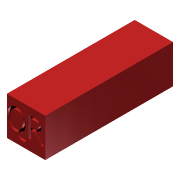
# Autodesk Inventor part: Container 2 2 5 QR color 5
Saved by Autodesk Inventor 2015 (Build 190159000, 159)
## iProperties
Created: 2015-03-07
Part Number: Container 2 2 5 QR color 5
Material: Generic
Document SubType Name: Modeling
Designer: Vukica
Density: 1 g/cm^3
Appearance: Light Red
Author: Vukica
Autodesk Inventor part; units mm, degrees
ref_plane "YZ Plane" through (0, 0, 0) normal (1, 0, 0) x (0, 1, 0)
ref_plane "XZ Plane" through (0, 0, 0) normal (0, 1, 0) x (-1, 0, 0)
ref_plane "XY Plane" through (0, 0, 0) normal (0, 0, 1) x (1, 0, 0)
sketch "Sketch1" plane through (0, 0, 0) normal (0, 0, 1) x (1, 0, 0)
  line L0 (0, 0) -> (38.1, 0)
  line L1 (38.1, 0) -> (38.1, 38.1)
  line L2 (38.1, 38.1) -> (0, 38.1)
  line L3 (0, 38.1) -> (0, 0)
  dimension "d0" = 38.1
  dimension "d1" = 38.1
  constraints: 8 end point, 2 parallel, 1 horizontal, 1 perpendicular
  measures "d0" distance of L1.end L2.end
  measures "d1" distance of L2.end L0.start
extrude "Extrusion1" add sketch "Sketch1" along normal blind 127
sketch "Sketch2" plane through (0, 0, 127) normal (0, 0, 1) x (1, 0, 0)
  line L0 (-0.4591, 31.2765) -> (45.936, 31.2765) construction
  line L1 (45.936, 31.2765) -> (45.936, -1.3483) construction
  line L2 (45.936, -1.3483) -> (-0.4591, -1.3483) construction
  line L3 (-0.4591, -1.3483) -> (-0.4591, 31.2765) construction
  spline S0 degree 2 poles (18.4777, 5.5554) (17.7367, 5.3742) (16.1229, 5.1766) (15.3161, 5.1766) knots 0 0 0 1 2 2 2
  spline S1 degree 2 poles (15.3161, 5.1766) (13.0272, 5.1766) (10.1784, 7.729) (10.0467, 10.1002) knots 0 0 0 1 2 2 2
  spline S2 degree 2 poles (10.0467, 10.1002) (9.8656, 10.1002) (9.5527, 10.1002) (9.421, 10.1002) knots 0 0 0 1 2 2 2
  spline S3 degree 2 poles (9.421, 10.1002) (7.3626, 10.1002) (4.0528, 11.4999) (2.8672, 12.8666) knots 0 0 0 1 2 2 2
  spline S4 degree 2 poles (2.8672, 12.8666) (1.698, 14.2169) (0.4466, 18.1689) (0.4466, 20.6719) knots 0 0 0 1 2 2 2
  spline S5 degree 2 poles (0.4466, 20.6719) (0.4466, 23.2407) (1.7145, 27.1269) (2.8837, 28.5101) knots 0 0 0 1 2 2 2
  spline S6 degree 2 poles (2.8837, 28.5101) (4.0693, 29.8768) (7.3791, 31.2765) (9.421, 31.2765) knots 0 0 0 1 2 2 2
  spline S7 degree 2 poles (9.421, 31.2765) (11.4958, 31.2765) (14.8221, 29.8274) (15.9747, 28.5101) knots 0 0 0 1 2 2 2
  spline S8 degree 2 poles (15.9747, 28.5101) (17.1274, 27.1763) (18.4118, 23.2078) (18.4118, 20.6719) knots 0 0 0 1 2 2 2
  spline S9 degree 2 poles (18.4118, 20.6719) (18.4118, 16.7198) (15.3325, 11.5822) (12.6485, 10.6765) knots 0 0 0 1 2 2 2
  spline S10 degree 2 poles (12.6485, 10.6765) (12.7143, 9.9191) (13.1095, 8.7005) (13.4224, 8.3547) knots 0 0 0 1 2 2 2
  spline S11 degree 2 poles (13.4224, 8.3547) (13.8011, 7.9266) (14.8385, 7.5314) (15.7607, 7.5314) knots 0 0 0 1 2 2 2
  spline S12 degree 2 poles (15.7607, 7.5314) (16.3041, 7.5314) (17.7861, 7.8772) (18.1154, 8.0089) knots 0 0 0 1 2 2 2
  line L4 (18.1154, 8.0089) -> (18.4777, 8.0089)
  line L5 (18.4777, 8.0089) -> (18.4777, 5.5554)
  spline S13 degree 2 poles (15.596, 20.6719) (15.596, 22.6973) (14.7233, 25.8095) (13.9329, 26.8304) knots 0 0 0 1 2 2 2
  spline S14 degree 2 poles (13.9329, 26.8304) (13.126, 27.8843) (10.8536, 28.9382) (9.4374, 28.9382) knots 0 0 0 1 2 2 2
  spline S15 degree 2 poles (9.4374, 28.9382) (7.9719, 28.9382) (5.7653, 27.9173) (4.9255, 26.8304) knots 0 0 0 1 2 2 2
  spline S16 degree 2 poles (4.9255, 26.8304) (4.1187, 25.793) (3.2624, 22.6479) (3.2624, 20.6719) knots 0 0 0 1 2 2 2
  spline S17 degree 2 poles (3.2624, 20.6719) (3.2624, 16.6704) (6.6216, 12.4056) (9.4374, 12.4056) knots 0 0 0 1 2 2 2
  spline S18 degree 2 poles (9.4374, 12.4056) (12.2532, 12.4056) (15.596, 16.6704) (15.596, 20.6719) knots 0 0 0 1 2 2 2
  line L6 (37.1016, 10.5283) -> (33.5942, 10.5283)
  line L7 (33.5942, 10.5283) -> (27.1721, 18.6135)
  line L8 (27.1721, 18.6135) -> (24.0764, 18.6135)
  line L9 (24.0764, 18.6135) -> (24.0764, 10.5283)
  line L10 (24.0764, 10.5283) -> (21.3758, 10.5283)
  line L11 (21.3758, 10.5283) -> (21.3758, 30.8483)
  line L12 (21.3758, 30.8483) -> (26.6123, 30.8483)
  spline S19 degree 2 poles (26.6123, 30.8483) (28.3578, 30.8483) (30.7125, 30.4696) (31.7828, 29.778) knots 0 0 0 1 2 2 2
  spline S20 degree 2 poles (31.7828, 29.778) (32.8532, 29.0864) (34.0882, 26.9292) (34.0882, 25.332) knots 0 0 0 1 2 2 2
  spline S21 degree 2 poles (34.0882, 25.332) (34.0882, 23.109) (31.8158, 20.0955) (29.8727, 19.371) knots 0 0 0 1 2 2 2
  line L13 (29.8727, 19.371) -> (37.1016, 10.5283)
  spline S22 degree 2 poles (31.2724, 25.1179) (31.2724, 26.0071) (30.6466, 27.3739) (29.988, 27.8185) knots 0 0 0 1 2 2 2
  spline S23 degree 2 poles (29.988, 27.8185) (29.4116, 28.1972) (27.8802, 28.5101) (26.7605, 28.5101) knots 0 0 0 1 2 2 2
  line L14 (26.7605, 28.5101) -> (24.0764, 28.5101)
  line L15 (24.0764, 28.5101) -> (24.0764, 20.8695)
  line L16 (24.0764, 20.8695) -> (26.4476, 20.8695)
  spline S24 degree 2 poles (26.4476, 20.8695) (27.6168, 20.8695) (29.4775, 21.2811) (30.1197, 21.9233) knots 0 0 0 1 2 2 2
  spline S25 degree 2 poles (30.1197, 21.9233) (30.7125, 22.4832) (31.2724, 24.064) (31.2724, 25.1179) knots 0 0 0 1 2 2 2
  point P0 (0, 0)
  constraints: 2 other
extrude "Extrusion2" cut sketch "Sketch2" against normal blind 2.54
body "Solid1"
